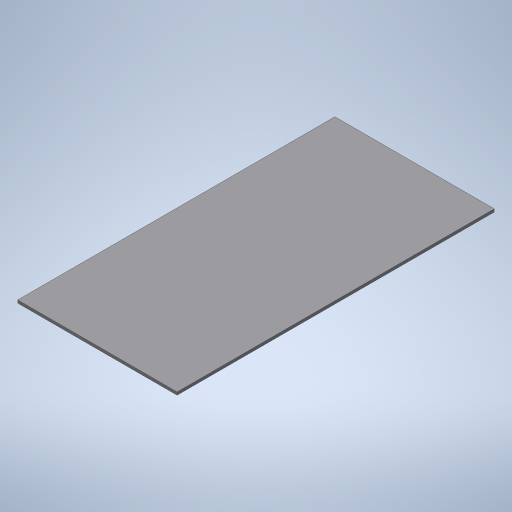
# Autodesk Inventor part: Door skeleton
Saved by Autodesk Inventor 2024 (Build 280153000, 153)
## iProperties
Created: 2014-10-21
Part Number: Door skeleton
Material: Generic
Document SubType Name: Modeling
Designer: G. Kazokaitis
Density: 1 g/cm^3
Appearance: Default
Author: G. Kazokaitis
Autodesk Inventor part; units mm, degrees
ref_plane "YZ Plane" through (0, 0, 0) normal (1, 0, 0) x (0, 1, 0)
ref_plane "XZ Plane" through (0, 0, 0) normal (0, 1, 0) x (-1, 0, 0)
ref_plane "XY Plane" through (0, 0, 0) normal (0, 0, 1) x (1, 0, 0)
sketch "Sketch2" plane through (0, 0, 0) normal (0, 0, 1) x (1, 0, 0)
  line L0 (-500, -1000) -> (500, -1000)
  line L1 (500, -1000) -> (500, 1000)
  line L2 (500, 1000) -> (-500, 1000)
  line L3 (-500, 1000) -> (-500, -1000)
  point P0 (0, 0)
  point P1 (0, 1000)
  point P2 (-500, 0)
  dimension "Door_width" = 1000
  dimension "Door_height" = 2000
  constraints: 8 end point, 2 midpoint, 2 parallel, 1 horizontal, 1 horizontal alignment, 1 perpendicular, 1 vertical alignment
  measures "Door_width" distance of L1.end L2.end
  measures "Door_height" distance between parallel lines of L0 L2
sketch "Sketch3" plane through (0, 0, 0) normal (0, 0, 1) x (1, 0, 0)
  line L0 (500, 1000) -> (-500, 1000) projected
  line L1 (-500, 1000) -> (-500, -1000) projected
  line L2 (500, -1000) -> (500, 1000) projected
  line L3 (-500, -1000) -> (500, -1000) projected
  line L4 (-500, 995) -> (500, 995)
  line L5 (500, 995) -> (500, -995)
  line L6 (500, -995) -> (-500, -995)
  line L7 (-500, -995) -> (-500, 995)
  point P0 (0, 0)
  dimension "d4" = 5
  dimension "d5" = 5
  constraints: 8 end point, 2 collinear, 2 parallel, 1 horizontal, 1 perpendicular
  measures "d4" distance between parallel lines of L0 L4
  measures "d5" distance between parallel lines of L3 L6
extrude "Extrusion1" add sketch "Sketch3" against normal blind 18 contours L2 L6 L1 L4
equation "\"d6\" = Board_Thickness"
equation "\"Board_Thickness\" = 18"
